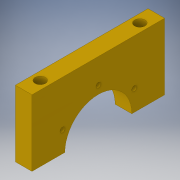
# Autodesk Inventor part: BottomOfSupportForAxel
Saved by Autodesk Inventor 2019.3 (Build 233278000, 278)
## iProperties
Created: 2019-01-06
Part Number: BottomOfSupportForAxel
Material: PBT Plastic
Document SubType Name: Modeling
Designer: steele
Density: 1.31 g/cm^3
Appearance: Gold
Author: steele
Autodesk Inventor part; units mm, degrees
ref_plane "YZ Plane" through (0, 0, 0) normal (1, 0, 0) x (0, 1, 0)
ref_plane "XZ Plane" through (0, 0, 0) normal (0, 1, 0) x (-1, 0, 0)
ref_plane "XY Plane" through (0, 0, 0) normal (0, 0, 1) x (1, 0, 0)
sketch "Sketch1" plane through (0, 0, 0) normal (1, 0, 0) x (0, 1, 0)
  line L0 (-25.4, -50.8) -> (25.4, -50.8)
  line L1 (25.4, -50.8) -> (25.4, 50.8)
  line L2 (25.4, 50.8) -> (-25.4, 50.8)
  line L3 (-25.4, 50.8) -> (25.4, -50.8) construction
  line L4 (-25.4, -50.8) -> (25.4, 50.8) construction
  arc A0 (-25.4, -25.654) -> (-25.4, 25.654) centre (-25.4, 0) ccw
  line L5 (-25.4, 50.8) -> (-25.4, 25.654)
  line L6 (-25.4, -25.654) -> (-25.4, -50.8)
  point P0 (0, 0)
  dimension "d0" = 101.6
  dimension "d1" = 50.8
  dimension "d2" = 51.308
  dimension "d6" = 50.8
  dimension "d7" = 50.8
  constraints: 14 end point, 3 parallel, 2 midpoint, 2 perpendicular, 2 point on circle, 1 centre point, 1 vertical
  measures "d0" distance of L0.end L1.end
  measures "d1" distance of L1.end L2.end
  measures "d2" diameter of A0
  measures "d6" distance from line of L1 A0.centre
  measures "d7" distance from line of L2 A0.centre
extrude "Extrusion1" add sketch "Sketch1" along normal mid plane 12.7
sketch "Sketch3" plane through (6.35, 0, 0) normal (1, 0, 0) x (0, 0, -1)
  circle A0 centre (0, -25.4) radius 31.75 construction
  point P0 (0, 0)
  point P1 (0, 6.35)
  point P2 (0, 6.35)
  point P3 (-27.4963, -9.525)
  point P4 (-27.4963, -41.275)
  point P5 (0, -57.15)
  point P6 (27.4963, -41.275)
  point P7 (27.4963, -9.525)
  dimension "d17" = 360
  constraints: 3 coincident, 1 centre point, 11 other
hole "Hole2" at (6.35, 6.35, 0) at (6.35, -9.525, 27.4963) at (6.35, -41.275, 27.4963) at (6.35, -57.15, 0) at (6.35, -41.275, -27.4963) at (6.35, -9.525, -27.4963) direction (-1, 0, 0) diameter 3.81 end through all clearance for "Flat Head Machine Screw (82)" size "#6" standard "Ansi Unified Screw Threads"
sketch "Sketch4" plane through (-6.35, 25.4, 50.8) normal (0, 1, 0) x (1, 0, 0)
  line L0 (12.7, 0) -> (0, 0) construction
  line L1 (6.35, 0) -> (6.35, 101.6) construction
  line L2 (12.7, 101.6) -> (0, 101.6) construction
  point P0 (6.35, 50.8)
  point P1 (6.35, 12.7)
  point P2 (6.35, 88.9)
  dimension "d26" = 12.7
  dimension "d27" = 12.7
  constraints: 2 end point, 2 midpoint, 2 point on line
  measures "d26" distance from line of L0 point (6.35, 12.7)
  measures "d27" distance from line of point (6.35, 88.9) L2
hole "Hole3" at (0, 25.4, 38.1) at (0, 25.4, -38.1) direction (0, -1, 0) diameter 6.7564 end through all clearance for "Flat Head Machine Screw (82)" size "1/4" standard "Ansi Unified Screw Threads"
sketch "Sketch5" plane through (-6.35, 25.4, 50.8) normal (0, 1, 0) x (1, 0, 0)
  circle A0 centre (6.35, 88.9) radius 3.3782 projected
  circle A1 centre (6.35, 88.9) radius 4.0132
  circle A2 centre (6.35, 12.7) radius 3.3782 projected
  circle A3 centre (6.35, 12.7) radius 4.0132
  point P0 (6.35, 50.8)
  dimension "d35" = 8.0264
  constraints: 2 centre point, 2 coincident, 1 equal radius
  measures "d35" diameter of A1
extrude "Extrusion2" cut sketch "Sketch5" against normal blind 12.7
body "Solid1"
